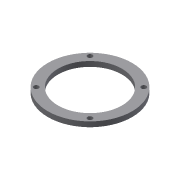
# Autodesk Inventor part: chamberPlateCircle
Saved by Autodesk Inventor 2013 (Build 170138000, 138)
## iProperties
Created: 2016-06-27
Part Number: chamberPlateCircle
Material: Generic
Document SubType Name: Modeling
Designer: 120pa
Density: 1 g/cm^3
Author: 120pa
Autodesk Inventor part; units mm, degrees
ref_plane "YZ Plane" through (0, 0, 0) normal (1, 0, 0) x (0, 1, 0)
ref_plane "XZ Plane" through (0, 0, 0) normal (0, 1, 0) x (-1, 0, 0)
ref_plane "XY Plane" through (0, 0, 0) normal (0, 0, 1) x (1, 0, 0)
sketch "Sketch1" plane through (0, 0, 0) normal (0, 1, 0) x (-1, 0, 0)
  circle A0 centre (0, 0) radius 19
  circle A1 centre (0, 0) radius 25
  dimension "d0" = 38
  dimension "d1" = 50
  constraints: 2 centre point
  measures "d0" diameter of A0
  measures "d1" diameter of A1
extrude "Extrusion1" add sketch "Sketch1" along normal blind 3
sketch "Sketch4" plane through (0, 3, 0) normal (0, 1, 0) x (1, 0, 0)
  line L0 (-16, -16) -> (16, -16)
  line L1 (16, -16) -> (16, 16)
  line L2 (16, 16) -> (-16, 16)
  line L3 (-16, 16) -> (-16, -16)
  line L4 (-16, -16) -> (16, 16) construction
  line L5 (16, -16) -> (-16, 16) construction
  point P0 (0, 0)
  dimension "d13" = 32
  dimension "d14" = 32
  constraints: 12 end point, 2 midpoint
  measures "d13" distance of L2.end L1.end
  measures "d14" distance of L1.end L0.end
hole "Hole2" at (-16, 3, 16) at (-16, 3, -16) at (16, 3, -16) at (16, 3, 16) direction (0, -1, 0) diameter 2.9 depth 8 tip angle 118 clearance for "Flat Head Machine Screw" size "M2.5" standard "Ansi Metric M Profile"
body "Solid1"
